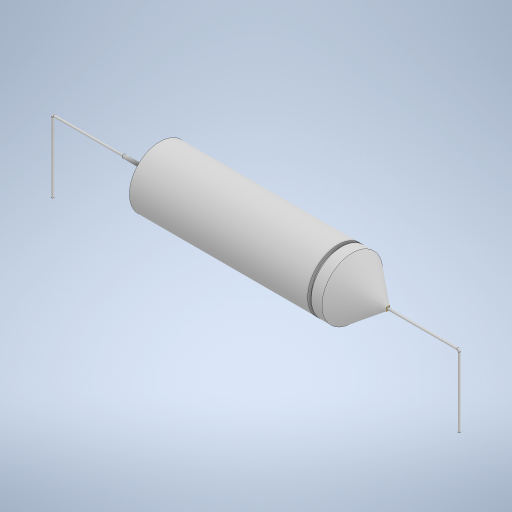
# Autodesk Inventor part: K50-29
Saved by Autodesk Inventor 2024 (Build 280153000, 153)
## iProperties
Created: 2023-12-14
Part Number: K50-29
Material: Generic
Document SubType Name: Sheet Metal
Designer: user
Density: 1 g/cm^3
Sheet Metal Rule: Default
Appearance: Default
Author: user
Autodesk Inventor part; units mm, degrees
ref_plane "YZ Plane" through (0, 0, 0) normal (1, 0, 0) x (0, 1, 0)
ref_plane "XZ Plane" through (0, 0, 0) normal (0, 1, 0) x (-1, 0, 0)
ref_plane "XY Plane" through (0, 0, 0) normal (0, 0, 1) x (1, 0, 0)
sketch "Sketch1" plane through (0, 0, 0) normal (0, 0, 1) x (1, 0, 0)
  line L0 (-18.5, 0) -> (-18.5, 0.25)
  line L1 (-18.5, 0.25) -> (-13.5, 0.25)
  line L2 (-13.5, 0.25) -> (-13.5, 4.25)
  line L3 (-13.5, 4.25) -> (11.5, 4.25)
  line L4 (11.5, 4.25) -> (11.5, 3.75)
  line L5 (11.5, 3.75) -> (12, 3.75)
  line L6 (12, 3.75) -> (12, 4.25)
  line L7 (12, 4.25) -> (13.5, 4.25)
  line L8 (18.5, 0) -> (18.5, 0.25)
  line L9 (18.5, 0.25) -> (13.5, 4.25)
  line L10 (18.5, 0) -> (-18.5, 0)
  point P0 (0, 0)
  dimension "d0" = 0.25
  dimension "d1" = 5
  dimension "d2" = 4
  dimension "d8" = 25
  dimension "d9" = 0.5
  dimension "d10" = 0.5
  dimension "d11" = 0.5
  dimension "d12" = 1.5
  dimension "d14" = 0.25
  constraints: 22 end point, 4 perpendicular, 2 horizontal, 2 point on line, 1 vertical
  measures "d0" distance of L0.start L0.end
  measures "d1" distance of L0.end L1.end
  measures "d2" distance of L1.end L2.end
  measures "d8" distance of L2.end L3.end
  measures "d9" distance of L3.end L4.end
  measures "d10" distance of L4.end L5.end
  measures "d11" distance of L5.end L6.end
  measures "d12" distance of L6.end L7.end
  measures "d14" distance of L8.start L8.end
revolve "Revolution1" add sketch "Sketch1" angle 360 about axis through (18.5, 0, 0) along (-1, 0, 0)
sketch "Sketch2" plane through (0, 0, 0) normal (0, 0, 1) x (1, 0, 0)
  line L0 (18.5, 0.25) -> (18.5, -0.25) projected
  line L1 (18.5, 0) -> (28.3, 0)
  line L2 (28.5, -0.2) -> (28.5, -10)
  arc A0 (28.5, -0.2) -> (28.3, 0) centre (28.3, -0.2) ccw
  point P0 (0, 0)
  point P1 (28.5, 0)
  dimension "d16" = 10
  dimension "d17" = 10
  dimension "d18" = 0.2
  constraints: 4 end point, 2 point on circle, 2 point on line, 2 tangent, 1 centre point, 1 horizontal, 1 midpoint, 1 perpendicular
  measures "d16" distance of L1.start point (28.5, 0)
  measures "d17" distance of point (28.5, 0) L2.end
  measures "d18" radius of A0
ref_plane "Work Plane1" through (18.5, 0, 0) normal (1, 0, 0) x (0, 0, -1)
sketch "Sketch3" plane through (18.5, 0, 0) normal (1, 0, 0) x (0, 0, -1)
  circle A0 centre (0, 0) radius 0.15
  dimension "d20" = 0.3
  constraints: 1 centre point, 1 coincident
  measures "d20" diameter of A0
sweep "Sweep1" add profiles "Sketch3" path "Sketch2" path curves L1 A0 L2
mirror "Mirror1" about plane through (0, 0, 0) normal (1, 0, 0) of "Sweep1"
equation "\"BendRadius\" = Thickness"
equation "\"BendReliefWidth\" = Thickness"
equation "\"BendReliefDepth\" = 0.5 * Thickness"
equation "\"CornerReliefSize\" = 4 * Thickness"
equation "\"MinimumRemnant\" = 2 * Thickness"
equation "\"TransitionRadius\" = BendRadius"
equation "\"JacobiRadiusSize\" = BendRadius"
equation "\"GapSize\" = Thickness"
equation "\"Thickness\" = 3.048"
body "Solid1"
